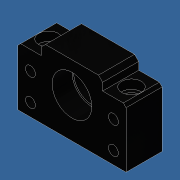
# Autodesk Inventor part: BF10 BEARING BLOCK
Saved by Autodesk Inventor 2013 SP1 (Build 170176100, 176)
## iProperties
Created: 2013-04-30
Part Number: BF10 BEARING BLOCK
Material: Aluminum 6061
Document SubType Name: Modeling
Designer: J.WASSERSTRASS
Mass: 87.0675 g
Surface Area: 108.551 cm^2
Volume: 32.1282 cm^3
Density: 2.71 g/cm^3
Author: J.WASSERSTRASS
Autodesk Inventor part; units mm, degrees
ref_plane "YZ Plane" through (0, 0, 0) normal (1, 0, 0) x (0, 1, 0)
ref_plane "XZ Plane" through (0, 0, 0) normal (0, 1, 0) x (-1, 0, 0)
ref_plane "XY Plane" through (0, 0, 0) normal (0, 0, 1) x (1, 0, 0)
sketch "Sketch1" plane through (0, 0, 0) normal (0, 0, 1) x (1, 0, 0)
  line L0 (0, 0) -> (-60, 0)
  line L1 (-60, 0) -> (-60, 32.5)
  line L2 (-60, 32.5) -> (0, 32.5)
  line L3 (0, 32.5) -> (0, 0)
  line L4 (-47, 39) -> (-13, 39)
  line L5 (-13, 39) -> (-13, 32.5)
  line L6 (-13, 32.5) -> (-47, 32.5)
  line L7 (-47, 32.5) -> (-47, 39)
  point P0 (-30, 32.5)
  dimension "d0" = 60
  dimension "d1" = 39
  dimension "d2" = 34
  dimension "d3" = 32.5
  constraints: 16 end point, 4 parallel, 2 horizontal, 2 midpoint, 2 perpendicular
  measures "d0" distance of L0.start L0.end
  measures "d1" distance between parallel lines of L0 L4
  measures "d2" distance of L4.start L4.end
  measures "d3" distance of L2.end L0.start
extrude "Extrusion1" add sketch "Sketch1" along normal blind 20
sketch "Sketch2" plane through (0, 0, 20) normal (0, 0, 1) x (1, 0, 0)
  line L0 (-13, 32.5) -> (-13, 39) projected
  line L1 (-13, 39) -> (-47, 39) projected
  line L2 (-47, 39) -> (-47, 32.5) projected
  line L3 (-47, 32.5) -> (-60, 32.5) projected
  line L4 (-60, 32.5) -> (-60, 0) projected
  line L5 (-60, 0) -> (0, 0) projected
  line L6 (0, 0) -> (0, 32.5) projected
  line L7 (0, 32.5) -> (-13, 32.5) projected
  line L8 (-30, 0) -> (-30, 22) construction
  dimension "d6" = 22
  constraints: 2 end point, 1 coincident, 1 midpoint, 1 perpendicular
  measures "d6" distance from line of point (-30, 22) L5
hole "Hole1" at (-30, 22, 20) direction (0, 0, -1) diameter 20 end through all counterbore diameter 22 counterbore depth 11
sketch "Sketch3" plane through (0, 0, 20) normal (0, 0, 1) x (1, 0, 0)
  circle A0 centre (-30, 22) radius 11 construction
  line L0 (-13, 32.5) -> (-13, 39) construction
  line L1 (-13, 39) -> (-47, 39) construction
  line L2 (-47, 39) -> (-47, 32.5) construction
  line L3 (-47, 32.5) -> (-60, 32.5) construction
  line L4 (-60, 32.5) -> (-60, 0) construction
  line L5 (-60, 0) -> (0, 0) construction
  line L6 (0, 0) -> (0, 32.5) construction
  line L7 (0, 32.5) -> (-13, 32.5) construction
  line L8 (-53, 22) -> (-7, 22) construction
  line L9 (-7, 22) -> (-7, 7) construction
  line L10 (-7, 7) -> (-53, 7) construction
  line L11 (-53, 7) -> (-53, 22) construction
  dimension "d14" = 15
  dimension "d16" = 46
  constraints: 8 end point, 5 coincident, 2 parallel, 1 horizontal, 1 midpoint, 1 perpendicular
  measures "d14" distance of L8.end L9.end
  measures "d16" distance of L9.end L10.end
hole "Hole2" at (-7, 22, 20) at (-7, 7, 20) at (-53, 22, 20) at (-53, 7, 20) direction (0, 0, -1) diameter 5.5 end through all
sketch "Sketch4" plane through (-60, 32.5, 0) normal (0, 1, 0) x (1, 0, 0)
  line L0 (13, 0) -> (13, -20) construction
  line L1 (13, 0) -> (0, 0) construction
  line L2 (0, 0) -> (0, -20) construction
  line L3 (13, -20) -> (0, -20) construction
  line L4 (47, 0) -> (47, -20) construction
  line L5 (60, -20) -> (47, -20) construction
  line L6 (60, 0) -> (60, -20) construction
  line L7 (60, 0) -> (47, 0) construction
  line L8 (60, -10) -> (53, -10) construction
  line L9 (0, -10) -> (7, -10) construction
  dimension "d24" = 46
  constraints: 4 end point, 2 coincident, 2 collinear, 2 midpoint, 1 parallel
  measures "d24" distance of point (7, -10) point (53, -10)
hole "Hole3" at (-53, 32.5, 10) at (-7, 32.5, 10) direction (0, -1, 0) diameter 6.6 end through all counterbore diameter 10.8 counterbore depth 5
chamfer "Chamfer1" distance 2.286 angle 45 2 edges at (-47, 39, 10) (-13, 39, 10)
chamfer "Chamfer2" distance 1.524 angle 45 2 edges at (-60, 32.5, 10) (0, 32.5, 10)
body "Solid1"
